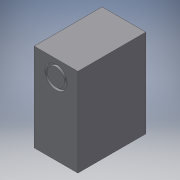
# Autodesk Inventor part: aqisensor
Saved by Autodesk Inventor 2019 (Build 230136000, 136)
## iProperties
Created: 2019-06-25
Part Number: aqisensor
Material: Generic
Document SubType Name: Modeling
Designer: Daniel
Density: 1 g/cm^3
Appearance: Default
Author: Daniel
Autodesk Inventor part; units mm, degrees
ref_plane "YZ Plane" through (0, 0, 0) normal (1, 0, 0) x (0, 1, 0)
ref_plane "XZ Plane" through (0, 0, 0) normal (0, 1, 0) x (-1, 0, 0)
ref_plane "XY Plane" through (0, 0, 0) normal (0, 0, 1) x (1, 0, 0)
sketch "Sketch1" plane through (0, 0, 0) normal (1, 0, 0) x (0, 1, 0)
  line L0 (0, 0) -> (46.1137, 0)
  line L1 (46.1137, 0) -> (46.1137, -35.56)
  line L2 (46.1137, -35.56) -> (0, -35.56)
  line L3 (0, -35.56) -> (0, 0)
  dimension "d0" = 46.1137
  dimension "d1" = 35.56
  constraints: 8 end point, 2 parallel, 1 horizontal, 1 perpendicular
  measures "d0" distance of L1.end L2.end
  measures "d1" distance of L0.end L1.end
extrude "Extrusion1" add sketch "Sketch1" along normal blind 22.86
sketch "Sketch2" plane through (0, 0, 0) normal (0, 0, 1) x (1, 0, 0)
  circle A0 centre (11.43, 37.8108) radius 5.8364
  circle A1 centre (11.43, 37.8108) radius 4.5919
  point P0 (0, 0)
  constraints: 2 centre point, 1 coincident
extrude "Extrusion2" cut sketch "Sketch2" against normal blind 1.27
scale "Scale1" factors (0.7, 0.7, 0.7) then translate (0, 6.9171, -5.334) bodies 1
body "Solid1"
